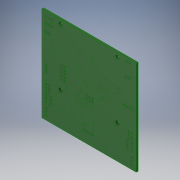
# Autodesk Inventor part: Kama-Sterownik-v1.brd_Outline
Saved by Autodesk Inventor 2019 (Build 230136000, 136)
## iProperties
Created: 2019-05-02
Part Number: Kama-Sterownik-v1.brd_Outline
Material: Generic
Document SubType Name: Modeling
Designer: John
Density: 1 g/cm^3
Appearance: Board Outline
Mass: 10.0901 g
Surface Area: 136.97 cm^2
Volume: 10.0901 cm^3
Author: John
Autodesk Inventor part; units mm, degrees
ref_plane "YZ Plane" through (0, 0, 0) normal (1, 0, 0) x (0, 1, 0)
ref_plane "XZ Plane" through (0, 0, 0) normal (0, 1, 0) x (-1, 0, 0)
ref_plane "XY Plane" through (0, 0, 0) normal (0, 0, 1) x (1, 0, 0)
sketch "Sketch1" plane through (0, 0, 0) normal (0, 0, 1) x (1, 0, 0)
  line L0 (0, 0) -> (80, 0)
  line L1 (80, 0) -> (80, 80)
  line L2 (80, 80) -> (0, 80)
  line L3 (0, 80) -> (0, 0)
  circle A0 centre (3.81, 64.77) radius 0.51
  circle A1 centre (6.35, 64.77) radius 0.51
  circle A2 centre (3.81, 35.56) radius 0.51
  circle A3 centre (3.81, 38.1) radius 0.51
  circle A4 centre (3.81, 40.64) radius 0.51
  circle A5 centre (76.2, 21.59) radius 0.51
  circle A6 centre (73.66, 21.59) radius 0.51
  circle A7 centre (76.2, 24.13) radius 0.51
  circle A8 centre (73.66, 24.13) radius 0.51
  circle A9 centre (76.2, 26.67) radius 0.51
  circle A10 centre (73.66, 26.67) radius 0.51
  circle A11 centre (76.2, 3.81) radius 0.51
  circle A12 centre (76.2, 6.35) radius 0.51
  circle A13 centre (76.2, 8.89) radius 0.51
  circle A14 centre (76.2, 13.97) radius 0.51
  circle A15 centre (76.2, 16.51) radius 0.51
  circle A16 centre (76.2, 19.05) radius 0.51
  circle A17 centre (72.39, 13.97) radius 0.51
  circle A18 centre (72.39, 16.51) radius 0.51
  circle A19 centre (72.39, 19.05) radius 0.51
  circle A20 centre (3.81, 71.12) radius 0.51
  circle A21 centre (6.35, 71.12) radius 0.51
  circle A22 centre (8.89, 71.12) radius 0.51
  circle A23 centre (77.47, 44.45) radius 0.51
  circle A24 centre (74.93, 44.45) radius 0.51
  circle A25 centre (72.39, 44.45) radius 0.51
  circle A26 centre (69.85, 44.45) radius 0.51
  circle A27 centre (71.12, 65.79) radius 0.51
  circle A28 centre (73.66, 65.79) radius 0.51
  circle A29 centre (6.35, 21.59) radius 0.51
  circle A30 centre (3.81, 21.59) radius 0.51
  circle A31 centre (6.35, 24.13) radius 0.51
  circle A32 centre (3.81, 24.13) radius 0.51
  circle A33 centre (6.35, 26.67) radius 0.51
  circle A34 centre (3.81, 26.67) radius 0.51
  circle A35 centre (3.81, 3.81) radius 0.51
  circle A36 centre (3.81, 6.35) radius 0.51
  circle A37 centre (3.81, 8.89) radius 0.51
  circle A38 centre (3.81, 13.97) radius 0.51
  circle A39 centre (3.81, 16.51) radius 0.51
  circle A40 centre (3.81, 19.05) radius 0.51
  circle A41 centre (7.62, 13.97) radius 0.51
  circle A42 centre (7.62, 16.51) radius 0.51
  circle A43 centre (7.62, 19.05) radius 0.51
  circle A44 centre (38.1, 35.56) radius 0.51
  circle A45 centre (38.1, 33.02) radius 0.51
  circle A46 centre (40.64, 35.56) radius 0.51
  circle A47 centre (40.64, 33.02) radius 0.51
  circle A48 centre (43.18, 35.56) radius 0.51
  circle A49 centre (43.18, 33.02) radius 0.51
  circle A50 centre (19.27, 36.52) radius 0.51
  circle A51 centre (16.73, 36.52) radius 0.51
  circle A52 centre (19.27, 39.06) radius 0.51
  circle A53 centre (16.73, 39.06) radius 0.51
  circle A54 centre (19.27, 41.6) radius 0.51
  circle A55 centre (16.73, 41.6) radius 0.51
  circle A56 centre (19.27, 44.14) radius 0.51
  circle A57 centre (16.73, 44.14) radius 0.51
  circle A58 centre (19.27, 46.68) radius 0.51
  circle A59 centre (16.73, 46.68) radius 0.51
  circle A60 centre (3.81, 76.2) radius 0.51
  circle A61 centre (6.35, 76.2) radius 0.51
  circle A62 centre (8.89, 76.2) radius 0.51
  circle A63 centre (74.3, 77.09) radius 0.51
  circle A64 centre (71.76, 77.09) radius 0.51
  circle A65 centre (35.56, 8.89) radius 0.51
  circle A66 centre (38.1, 8.89) radius 0.51
  circle A67 centre (40.64, 8.89) radius 0.51
  circle A68 centre (43.18, 8.89) radius 0.51
  circle A69 centre (15.9, 76.6) radius 1.5
  circle A70 centre (64.1, 76.6) radius 1.5
  circle A71 centre (64.1, 28.4) radius 1.5
  circle A72 centre (15.9, 28.4) radius 1.5
  circle A73 centre (20.32, 27.94) radius 0.175
  circle A74 centre (33.274, 25.654) radius 0.175
  circle A75 centre (29.591, 25.654) radius 0.175
  circle A76 centre (42.418, 26.416) radius 0.175
  circle A77 centre (43.18, 28.321) radius 0.175
  circle A78 centre (43.18, 17.78) radius 0.175
  circle A79 centre (38.1, 41.91) radius 0.175
  circle A80 centre (12.192, 22.987) radius 0.175
  circle A81 centre (69.85, 27.94) radius 0.175
  circle A82 centre (57.912, 31.242) radius 0.175
  circle A83 centre (43.18, 31.2958) radius 0.175
  circle A84 centre (52.959, 46.99) radius 0.175
  circle A85 centre (50.673, 51.562) radius 0.175
  circle A86 centre (36.195, 45.212) radius 0.175
  circle A87 centre (20.32, 33.02) radius 0.175
  circle A88 centre (15.367, 73.66) radius 0.175
  circle A89 centre (8.89, 73.66) radius 0.175
  circle A90 centre (55.88, 8.89) radius 0.175
  circle A91 centre (55.88, 20.32) radius 0.175
  circle A92 centre (55.88, 39.37) radius 0.175
  circle A93 centre (53.34, 55.88) radius 0.175
  circle A94 centre (54.61, 48.514) radius 0.175
  circle A95 centre (30.48, 21.59) radius 0.175
  circle A96 centre (33.02, 6.35) radius 0.175
  circle A97 centre (33.274, 27.559) radius 0.175
  circle A98 centre (34.29, 17.78) radius 0.175
  circle A99 centre (49.53, 13.97) radius 0.175
  circle A100 centre (45.72, 7.62) radius 0.175
  circle A101 centre (44.831, 17.018) radius 0.175
  circle A102 centre (25.4, 21.59) radius 0.175
  circle A103 centre (25.908, 17.2184) radius 0.175
  circle A104 centre (33.02, 35.56) radius 0.175
  circle A105 centre (34.29, 52.07) radius 0.175
  circle A106 centre (31.75, 76.2) radius 0.175
  circle A107 centre (43.307, 76.2) radius 0.175
  circle A108 centre (51.816, 69.723) radius 0.175
  circle A109 centre (33.02, 66.04) radius 0.175
  circle A110 centre (43.18, 46.99) radius 0.175
  circle A111 centre (42.799, 61.976) radius 0.175
  circle A112 centre (64.389, 50.038) radius 0.175
  circle A113 centre (64.516, 46.228) radius 0.175
  circle A114 centre (10.16, 33.02) radius 0.175
  circle A115 centre (43.307, 66.167) radius 0.175
  circle A116 centre (43.307, 65.151) radius 0.175
  circle A117 centre (31.496, 64.643) radius 0.175
  circle A118 centre (16.51, 17.78) radius 0.175
  circle A119 centre (5.334, 11.811) radius 0.175
  circle A120 centre (8.128, 8.255) radius 0.175
  circle A121 centre (63.881, 14.605) radius 0.175
  circle A122 centre (50.8, 44.45) radius 0.175
  circle A123 centre (48.387, 43.815) radius 0.175
  circle A124 centre (30.734, 32.893) radius 0.175
  circle A125 centre (43.434, 12.319) radius 0.175
  circle A126 centre (36.957, 12.446) radius 0.175
  circle A127 centre (36.322, 13.589) radius 0.175
  circle A128 centre (43.434, 13.335) radius 0.175
  circle A129 centre (48.6128, 37.338) radius 0.175
  circle A130 centre (52.451, 39.243) radius 0.175
  circle A131 centre (49.403, 37.973) radius 0.175
  circle A132 centre (51.308, 40.894) radius 0.175
  circle A133 centre (50.927, 40.005) radius 0.175
  circle A134 centre (50.165, 38.608) radius 0.175
  circle A135 centre (43.434, 11.303) radius 0.175
  circle A136 centre (35.052, 11.938) radius 0.175
  circle A137 centre (43.434, 14.478) radius 0.175
  circle A138 centre (37.084, 14.478) radius 0.175
  circle A139 centre (39.243, 14.605) radius 0.175
  circle A140 centre (12.7, 29.845) radius 0.175
  circle A141 centre (75.946, 67.818) radius 0.35
  circle A142 centre (65.532, 54.483) radius 0.35
  circle A143 centre (38.608, 30.226) radius 0.175
  circle A144 centre (29.083, 31.242) radius 0.175
  circle A145 centre (39.6924, 29.337) radius 0.175
  circle A146 centre (29.972, 32.004) radius 0.175
  circle A147 centre (36.449, 30.226) radius 0.175
  circle A148 centre (29.718, 29.464) radius 0.175
  circle A149 centre (9.017, 60.833) radius 0.175
  circle A150 centre (9.017, 55.499) radius 0.175
  circle A151 centre (37.465, 30.226) radius 0.175
  circle A152 centre (29.845, 30.4236) radius 0.175
  circle A153 centre (36.4561, 28.3281) radius 0.175
  circle A154 centre (34.29, 30.734) radius 0.175
  circle A155 centre (54.356, 45.212) radius 0.175
  circle A156 centre (47.244, 45.212) radius 0.175
  circle A157 centre (36.1416, 27.3672) radius 0.175
  circle A158 centre (33.147, 30.734) radius 0.175
  circle A159 centre (50.927, 47.7746) radius 0.175
  circle A160 centre (48.768, 47.6476) radius 0.175
  constraints: 161 centre point, 8 end point
extrude "Kama Sterownik v1.brd_Outline" add sketch "Sketch1" along normal blind 1.6
body "Solid1"
